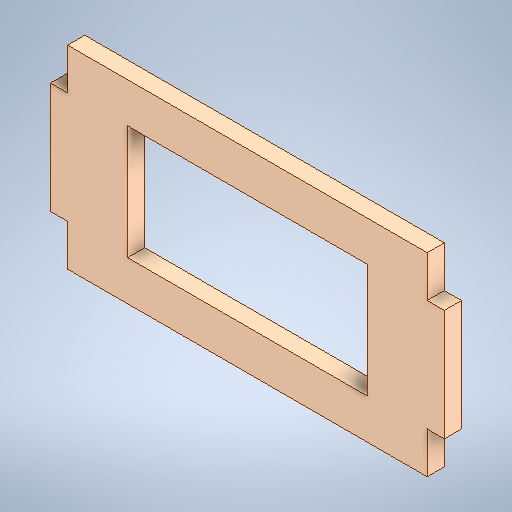
# Autodesk Inventor part: C
Saved by Autodesk Inventor 2025.3 (Build 293356030, 356C)
## iProperties
Created: 2025-07-09
Part Number: C
Material: Generic
Document SubType Name: Modeling
Designer: jv
Density: 1 g/cm^3
Appearance: Default(1)
Author: jv
Autodesk Inventor part; units mm, degrees
ref_plane "YZ Plane" through (0, 0, 0) normal (1, 0, 0) x (0, 1, 0)
ref_plane "XZ Plane" through (0, 0, 0) normal (0, 1, 0) x (-1, 0, 0)
ref_plane "XY Plane" through (0, 0, 0) normal (0, 0, 1) x (1, 0, 0)
sketch "Sketch1" plane through (0, 0, 0) normal (0, 0, 1) x (1, 0, 0)
  line L0 (-34.5, 17) -> (34.5, 17)
  line L1 (34.5, 17) -> (34.5, -17)
  line L2 (34.5, -17) -> (-34.5, -17)
  line L3 (-34.5, -17) -> (-34.5, 17)
  line L4 (34.5, 9.75) -> (31.5, 9.75)
  line L5 (31.5, 9.75) -> (31.5, -9.75)
  line L6 (31.5, -9.75) -> (34.5, -9.75)
  line L7 (34.5, -9.75) -> (34.5, 9.75)
  line L8 (-21, 10) -> (21, 10)
  line L9 (21, 10) -> (21, -10)
  line L10 (21, -10) -> (-21, -10)
  line L11 (-21, -10) -> (-21, 10)
  line L12 (0, 31.4058) -> (0, -31.4058)
  line L13 (31.5, 17) -> (31.5, 9.75)
  line L14 (31.5, -9.75) -> (31.5, -17)
  line L15 (-34.5, 17) -> (-34.5, -17)
  line L16 (-34.5, 9.75) -> (-31.5, 9.75)
  line L17 (-31.5, 9.75) -> (-31.5, -9.75)
  line L18 (-31.5, -9.75) -> (-34.5, -9.75)
  line L19 (-31.5, 17) -> (-31.5, 9.75)
  line L20 (-31.5, -9.75) -> (-31.5, -17)
  point P0 (0, 0)
  point P1 (34.5, 0)
  point P2 (0, 17)
  point P3 (34.5, 0)
  point P4 (21, 0)
  point P5 (0, 10)
  point P6 (-31, 17)
  point P7 (-31, -17)
  point P8 (31.5, -17)
  point P9 (0, 0)
  dimension "d0" = 34
  dimension "d1" = 19.5
  dimension "d2" = 3
  dimension "d3" = 20
  dimension "d4" = 69
  dimension "d5" = 42
  constraints: 42 end point, 8 point on line, 6 midpoint, 6 parallel, 6 symmetric about line, 3 horizontal, 3 horizontal alignment, 3 perpendicular, 2 vertical alignment, 1 coincident, 1 collinear, 1 vertical
  measures "d0" distance of L0.end L1.end
  measures "d1" distance of L4.end L5.end
  measures "d2" distance of L4.start L4.end
  measures "d3" distance of L8.end L9.end
  measures "d4" distance of L0.start L0.end
  measures "d5" distance of L8.start L8.end
extrude "Extrusion1" add sketch "Sketch1" along normal mid plane 3 contours L0 L12 L8 L11 L10 L2 L20 L17 L19 | L16 L17 L18 L3 | L0 L13 L5 L14 L2 L12 L10 L9 L8 | L4 L1 L6 L5
body "Solid1"
